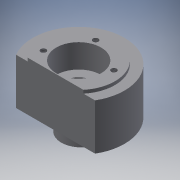
# Autodesk Inventor part: Ross Made spacer
Saved by Autodesk Inventor 2016 (Build 200138000, 138)
## iProperties
Created: 2017-07-25
Part Number: Ross Made spacer
Material: Generic
Document SubType Name: Modeling
Designer: M227562
Density: 1 g/cm^3
Appearance: Default
Author: M227562
Autodesk Inventor part; units mm, degrees
ref_plane "YZ Plane" through (0, 0, 0) normal (1, 0, 0) x (0, 1, 0)
ref_plane "XZ Plane" through (0, 0, 0) normal (0, 1, 0) x (-1, 0, 0)
ref_plane "XY Plane" through (0, 0, 0) normal (0, 0, 1) x (1, 0, 0)
sketch "Sketch1" plane through (0, 0, 0) normal (0, 0, 1) x (1, 0, 0)
  circle A0 centre (0, 0) radius 34.75
  dimension "d0" = 69.5
  constraints: 1 centre point, 1 coincident
  measures "d0" diameter of A0
extrude "Extrusion1" add sketch "Sketch1" along normal blind 35
sketch "Sketch2" plane through (0, 0, 35) normal (0, 0, 1) x (1, 0, 0)
  circle A0 centre (0, 0) radius 27.5
  dimension "d3" = 55
  constraints: 1 centre point, 1 coincident
  measures "d3" diameter of A0
extrude "Extrusion2" add sketch "Sketch2" along normal blind 2.5
sketch "Sketch3" plane through (0, 0, 37.5) normal (0, 0, 1) x (1, 0, 0)
  circle A0 centre (0, 0) radius 17
  dimension "d6" = 34
  constraints: 1 centre point, 1 coincident
  measures "d6" diameter of A0
extrude "Extrusion3" cut sketch "Sketch3" against normal blind 18
sketch "Sketch4" plane through (0, 0, 19.5) normal (0, 0, 1) x (1, 0, 0)
  circle A0 centre (0, 0) radius 9.85
  dimension "d9" = 19.7
  constraints: 1 centre point, 1 coincident
  measures "d9" diameter of A0
extrude "Extrusion4" cut sketch "Sketch4" against normal through all
sketch "Sketch5" plane through (0, 0, 0) normal (0, 0, -1) x (-1, 0, 0)
  circle A0 centre (0, 1.85) radius 15
  circle A1 centre (0, 0) radius 9.85 projected
  circle A2 centre (0, 0) radius 34.75 projected
  point P0 (0, -13.15)
  point P1 (0, -9.85)
  point P2 (0, 16.85)
  point P3 (0, 34.75)
  point P4 (0, 9.85)
  dimension "d12" = 30
  dimension "d13" = 3.3
  dimension "d14" = 7
  constraints: 4 point on circle, 1 centre point, 1 vertical alignment, 1 other
  measures "d12" diameter of A0
  measures "d13" distance of A1.start A0.start
  measures "d14" distance of A1.end A0.end
extrude "Extrusion5" add sketch "Sketch5" along normal blind 10 contours A0
sketch "Sketch6" plane through (0, 0, 0) normal (0, 0, -1) x (-1, 0, 0)
  circle A0 centre (0, 0) radius 34.75 projected
  line L0 (0, 34.75) -> (0, -17.55)
  line L1 (-32.813, -17.55) -> (43.7984, -17.55)
  line L2 (43.7984, -17.55) -> (43.7984, -45.8999)
  line L3 (43.7984, -45.8999) -> (-32.813, -45.8999)
  line L4 (-32.813, -45.8999) -> (-32.813, -17.55)
  dimension "d17" = 52.3
  constraints: 10 end point, 2 perpendicular, 1 horizontal, 1 vertical, 1 vertical alignment, 1 other
  measures "d17" distance of L0.start L0.end
extrude "Extrusion6" cut sketch "Sketch6" against normal through all contours L1 L2 L3 L4 A0 | A0 L1
sketch "Sketch7" plane through (0, 0, 37.5) normal (0, 0, 1) x (1, 0, 0)
  circle A0 centre (-6.9364, 19.8214) radius 2.25 projected
  circle A1 centre (19.8214, 6.9364) radius 2.25 projected
  circle A2 centre (-19.8214, -6.9364) radius 2.25 projected
  point P0 (0, 0)
  constraints: 3 coincident
hole "Hole1" at (-6.9364, 19.8214, 37.5) at (-19.8214, -6.9364, 37.5) at (19.8214, 6.9364, 37.5) direction (0, 0, -1) diameter 4.134 depth 14.2 tip angle 118 thread size "M5x0.8" class "6H" standard "ISO Metric profile"
body "Solid1"
